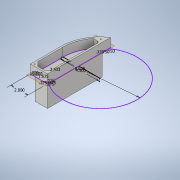
# Autodesk Inventor part: enclosure
Saved by Autodesk Inventor 2021 (Build 250183000, 183)
## iProperties
Created: 2020-11-08
Part Number: enclosure
Material: Generic
Document SubType Name: Modeling
Designer: mackeycj
Density: 1 g/cm^3
Appearance: Default
Author: mackeycj
Autodesk Inventor part; units mm, degrees
ref_plane "YZ Plane" through (0, 0, 0) normal (1, 0, 0) x (0, 1, 0)
ref_plane "XZ Plane" through (0, 0, 0) normal (0, 1, 0) x (-1, 0, 0)
ref_plane "XY Plane" through (0, 0, 0) normal (0, 0, 1) x (1, 0, 0)
sketch "Sketch1" plane through (0, 0, 0) normal (0, 1, 0) x (-1, 0, 0)
  arc A0 (63.5, -95.0381) -> (114.3, 0) centre (0, 0) ccw
  line L0 (114.3, 0) -> (114.3, 91.948)
  line L1 (114.3, 91.948) -> (63.5, 91.948)
  line L2 (63.5, 91.948) -> (63.5, -95.0381)
  arc A1 (68.2625, 85.6662) -> (109.5375, 0) centre (0, 0) ccw
  line L3 (109.5375, 0) -> (109.5375, 87.1855)
  line L4 (109.5375, 87.1855) -> (68.2625, 87.1855)
  line L5 (68.2625, 87.1855) -> (68.2625, -85.6662)
  line L6 (109.5375, 87.1855) -> (109.5375, 74.4855)
  line L7 (109.5375, 87.1855) -> (96.8375, 87.1855)
  line L8 (96.8375, 87.1855) -> (109.5375, 74.4855)
  line L9 (68.2625, 87.1855) -> (68.2625, 77.6605)
  line L10 (68.2625, 87.1855) -> (77.7875, 87.1855)
  line L11 (77.7875, 87.1855) -> (68.2625, 77.6605)
  line L12 (68.2625, -85.6662) -> (68.2625, -66.6162)
  line L13 (68.2625, -66.6162) -> (86.9526, -66.6162)
  line L14 (114.3, 91.948) -> (114.3, 85.598)
  line L15 (114.3, 85.598) -> (107.95, 85.598)
  line L16 (63.5, 91.948) -> (63.5, 84.963)
  line L17 (63.5, 84.963) -> (70.485, 84.963)
  line L18 (63.5, -95.0381) -> (63.5, -75.9881)
  line L19 (63.5, -75.9881) -> (73.025, -75.9881)
  dimension "d2" = 50.8
  dimension "d10" = 219.075
  dimension "d11" = 87.1855
  dimension "d13" = 41.275
  dimension "d14" = 12.7
  dimension "d15" = 12.7
  dimension "d16" = 9.525
  dimension "d17" = 9.525
  dimension "d18" = 19.05
  dimension "d19" = 6.35
  dimension "d20" = 6.35
  dimension "d21" = 6.985
  dimension "d22" = 6.985
  dimension "d23" = 19.05
  dimension "d24" = 9.525
  constraints: 40 end point, 9 point on line, 6 perpendicular, 6 point on circle, 2 centre point, 2 coincident, 2 horizontal, 2 tangent, 1 parallel, 1 vertical
  measures "d2" distance of L0.end L2.start
  measures "d10" diameter of A1
  measures "d11" distance of L3.start L3.end
  measures "d13" distance of L3.end L4.end
  measures "d14" distance of L3.end L6.end
  measures "d15" distance of L3.end L7.end
  measures "d16" distance of L4.end L9.end
  measures "d17" distance of L4.end L10.end
  measures "d18" distance of L5.end L12.end
  measures "d19" distance of L0.end L14.end
  measures "d20" distance of L14.end L15.end
  measures "d21" distance of L2.start L16.end
  measures "d22" distance of L16.end L17.end
  measures "d23" distance of L2.end L18.end
  measures "d24" distance of L18.end L19.end
extrude "Extrusion1" add sketch "Sketch1" along normal blind 25.4 contours L2 A1 L3 L15 L0 A0 | L2 L19 L5 A1 | L15 L3 L4 L5 A1 L2 L1 L0 | L2 L17 L5 L19 | A1 L5 L17 L2 | L5 L13 A1 | L3 L8 L4 | L5 L4 L11
ref_plane "Work Plane1" through (0, 0, 0) normal (0, 1, 0) x (1, 0, 0)
sketch "Sketch2" plane through (0, 0, 0) normal (0, 1, 0) x (1, 0, 0)
  line L0 (-114.3, -91.948) -> (-63.5, -91.948) projected
  line L1 (-77.7875, -87.1855) -> (-96.8375, -87.1855) projected
  line L2 (-63.5, -91.948) -> (-87.3125, -91.948)
  line L3 (-87.3125, -91.948) -> (-87.3125, -87.1855)
  line L4 (-87.3125, -87.1855) -> (-63.5, -87.1855)
  line L5 (-63.5, -87.1855) -> (-63.5, -91.948)
  line L6 (-68.2625, -77.6605) -> (-77.7875, -87.1855) projected
  line L7 (-77.7875, -87.1855) -> (-68.2625, -77.6605)
  circle A0 centre (-68.2625, -87.1855) radius 1.397 projected
  line L8 (-68.2625, -77.6605) -> (-68.2625, -87.1855)
  line L9 (-63.5, -91.948) -> (-63.5, 95.0381) projected
  line L10 (-68.2625, 66.6162) -> (-68.2625, -77.6605) projected
  line L11 (-63.5, -91.948) -> (-68.2625, -91.948)
  line L12 (-68.2625, -91.948) -> (-68.2625, 66.6162)
  line L13 (-68.2625, 66.6162) -> (-63.5, 66.6162)
  line L14 (-63.5, 66.6162) -> (-63.5, -91.948)
  line L15 (-63.5, 66.6162) -> (-76.2, 66.6162)
  line L16 (-76.2, 66.6162) -> (-76.2, 69.7912)
  line L17 (-76.2, 69.7912) -> (-63.5, 69.7912)
  line L18 (-63.5, 69.7912) -> (-63.5, 66.6162)
  line L19 (-114.3, -91.948) -> (-63.5, -91.948) projected
  line L20 (-114.3, -91.948) -> (-87.3125, -91.948)
  line L21 (-87.3125, -91.948) -> (-87.3125, -87.1855)
  line L22 (-87.3125, -87.1855) -> (-100.0125, -87.1855)
  line L23 (-100.0125, -87.1855) -> (-100.0125, -91.948)
  line L24 (-100.0125, -91.948) -> (-87.3125, -91.948)
  line L25 (-87.3125, -91.948) -> (-87.3125, -87.1855)
  point P0 (0, 0)
  point P1 (-87.3125, -91.948)
  point P2 (-68.2625, -85.7885)
  point P3 (-69.6595, -87.1855)
  dimension "d35" = 23.8125
  dimension "d36" = 12.7
  dimension "d37" = 3.175
  dimension "d58" = 12.7
  constraints: 40 end point, 9 equal length, 4 horizontal, 4 perpendicular, 1 midpoint, 1 point on line, 1 vertical
  measures "d35" distance of L3.end L4.end
  measures "d36" distance of L16.end L17.end
  measures "d37" distance of L15.end L16.end
  measures "d58" distance of L24.end L23.end
hole "Hole2" at (-107.95, 0, 85.598) at (-73.025, 0, -75.9881) direction (0, 1, 0) diameter 3.2766 end through all clearance for "Flat Head Machine Screw (82)" size "#4" standard "Ansi Unified Screw Threads"
extrude "Extrusion2" add sketch "Sketch2" against normal blind 63.5 contours L23 L22 L1 L3 L0 | L3 L1 L4 A0 L12 L0 | L12 A0 L4 L5 L0 | L12 L4 A0 | A0 L4 L12 | L4 A0 L8 L10 L13 L9 | L4 L8 A0 | L13 L15 L16 L17 L9 picked at (-67.389, -86.8798)
sketch "Sketch3" plane through (0, 0, 0) normal (0, 1, 0) x (-1, 0, 0)
  line L0 (104.775, 82.423) -> (111.125, 82.423)
  line L1 (111.125, 82.423) -> (111.125, 88.773)
  line L2 (111.125, 88.773) -> (104.775, 88.773)
  line L3 (104.775, 88.773) -> (104.775, 82.423)
  circle A0 centre (107.95, 85.598) radius 1.6383 projected
  line L4 (104.775, 82.423) -> (111.125, 88.773) construction
  line L5 (111.125, 82.423) -> (104.775, 88.773) construction
  line L6 (69.85, -79.1631) -> (76.2, -79.1631)
  line L7 (76.2, -79.1631) -> (76.2, -72.8131)
  line L8 (76.2, -72.8131) -> (69.85, -72.8131)
  line L9 (69.85, -72.8131) -> (69.85, -79.1631)
  circle A1 centre (73.025, -75.9881) radius 1.6383 projected
  line L10 (69.85, -79.1631) -> (76.2, -72.8131) construction
  line L11 (76.2, -79.1631) -> (69.85, -72.8131) construction
  point P0 (0, 0)
  dimension "d47" = 6.35
  dimension "d48" = 6.35
  dimension "d49" = 6.35
  dimension "d50" = 6.35
  constraints: 24 end point, 4 midpoint, 4 parallel, 2 horizontal, 2 perpendicular
  measures "d47" distance of L2.end L1.end
  measures "d48" distance of L1.end L0.end
  measures "d49" distance of L8.end L7.end
  measures "d50" distance of L7.end L6.end
extrude "Extrusion3" cut sketch "Sketch3" along normal blind 3.175
fillet "Fillet3" radius 12.7 1 edges at (-76.2, 0, -68.2037)
sketch "Sketch4" plane through (0, 0, 0) normal (0, 0, 1) x (1, 0, 0)
  line L0 (0, 0) -> (-114.3, 0)
  line L1 (-109.5375, 0) -> (-88.9, 0) projected
  dimension "d57" = 114.3
  constraints: 2 end point, 1 collinear
  measures "d57" distance of L0.start L0.end
fillet "Fillet4" radius 6.35 1 edges at (-68.2625, -31.75, 87.1855)
fillet "Fillet5" radius 6.35 1 edges at (-68.2625, -19.05, -66.6162)
body "Solid1"
